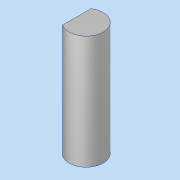
# Autodesk Inventor part: Encoder Shaft
Saved by Autodesk Inventor 2017 SP1 (Build 210196100, 196)
## iProperties
Created: 2018-12-30
Part Number: Encoder Shaft
Material: Aluminum 6061
Document SubType Name: Modeling
Designer: Dylan Rice
Density: 2.7 g/cm^3
Appearance: Aluminum - Flat
Author: Dylan Rice
Autodesk Inventor part; units mm, degrees
ref_plane "YZ Plane" through (0, 0, 0) normal (1, 0, 0) x (0, 1, 0)
ref_plane "XZ Plane" through (0, 0, 0) normal (0, 1, 0) x (-1, 0, 0)
ref_plane "XY Plane" through (0, 0, 0) normal (0, 0, 1) x (1, 0, 0)
sketch "Sketch1" plane through (0, 0, 0) normal (0, 1, 0) x (-1, 0, 0)
  arc A0 (0.8292, 1.25) -> (0.8292, -1.25) centre (0, 0) ccw
  line L0 (0.8292, 1.25) -> (0.8292, -1.25)
  dimension "d0" = 3
  dimension "d1" = 2.5
  constraints: 2 end point, 2 point on circle, 1 centre point, 1 coincident, 1 vertical
  measures "d0" diameter of A0
  measures "d1" distance of L0.start L0.end
extrude "Extrusion1" add sketch "Sketch1" along normal blind 10
body "Solid1"
